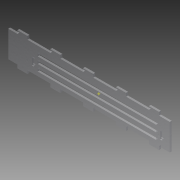
# Autodesk Inventor part: Panel3
Saved by Autodesk Inventor 2015 SP1 (Build 190203100, 203)
## iProperties
Created: 2014-08-06
Part Number: Panel3
Material: Acrylic, Clear
Document SubType Name: Modeling
Designer: Patrick Camilleri
Density: 1.19 g/cm^3
Appearance: Transparent - Clear
Author: Patrick Camilleri
Autodesk Inventor part; units mm, degrees
ref_plane "YZ Plane" through (0, 0, 0) normal (1, 0, 0) x (0, 1, 0)
ref_plane "XZ Plane" through (0, 0, 0) normal (0, 1, 0) x (-1, 0, 0)
ref_plane "XY Plane" through (0, 0, 0) normal (0, 0, 1) x (1, 0, 0)
sketch "Sketch1" plane through (0, 0, 0) normal (0, 1, 0) x (-1, 0, 0)
  line L0 (20.15, 134.75) -> (-20.15, 134.75)
  line L1 (-20.15, 134.75) -> (-20.15, -110.95)
  line L2 (-20.15, -110.95) -> (20.15, -110.95)
  line L3 (20.15, -110.95) -> (20.15, 134.75)
  line L4 (20.15, 0) -> (-20.15, 0) construction
  line L5 (0, -110.95) -> (0, 134.75) construction
  point P0 (0, 0)
  point P1 (0, 0)
  dimension "d57" = 40.3
  dimension "d58" = 110.95
  dimension "d59" = 134.75
  constraints: 12 end point, 3 midpoint, 2 parallel, 2 perpendicular, 2 point on line, 1 coincident, 1 horizontal
  measures "d57" distance of L1.end L2.end
  measures "d58" distance between parallel lines of L4 L2
  measures "d59" distance between parallel lines of L4 L0
extrude "Extrusion1" add sketch "Sketch1" along normal blind 3
sketch "Sketch3" plane through (0, 0, 0) normal (0, -1, 0) x (1, 0, 0)
  line L0 (20.15, -110.95) -> (-20.15, -110.95) projected
  line L1 (20.15, 134.75) -> (20.15, -110.95) projected
  line L2 (-20.15, -110.95) -> (-20.15, 134.75) projected
  line L3 (-25.15, -79.15) -> (-20.15, -79.15)
  line L4 (-20.15, -79.15) -> (-20.15, -94.45)
  line L5 (-20.15, -94.45) -> (-25.15, -94.45)
  line L6 (-25.15, -94.45) -> (-25.15, -79.15)
  line L7 (-25.15, -79.15) -> (-20.15, -94.45) construction
  line L8 (-20.15, -79.15) -> (-25.15, -94.45) construction
  line L9 (25.15, -94.45) -> (20.15, -94.45)
  line L10 (20.15, -94.45) -> (20.15, -79.15)
  line L11 (20.15, -79.15) -> (25.15, -79.15)
  line L12 (25.15, -79.15) -> (25.15, -94.45)
  line L13 (25.15, -94.45) -> (20.15, -79.15) construction
  line L14 (20.15, -94.45) -> (25.15, -79.15) construction
  point P0 (0, 0)
  point P1 (-22.65, -86.8)
  point P2 (22.65, -86.8)
  point P3 (20.15, -86.8)
  dimension "d61" = 15.3
  dimension "d64" = 5
  dimension "d65" = 15.3
  dimension "d78" = 24.15
  dimension "d79" = 24.15
  dimension "d97" = 5
  constraints: 24 end point, 5 midpoint, 4 parallel, 2 horizontal, 2 perpendicular, 2 point on line
  measures "d61" distance of L3.end L4.end
  measures "d64" distance of L10.end L11.end
  measures "d65" distance of L9.end L10.end
  measures "d78" distance from line of L0 point (-22.65, -86.8)
  measures "d79" distance from line of L0 point (22.65, -86.8)
  measures "d97" distance between parallel lines of L6 L4
extrude "Extrusion3" add sketch "Sketch3" against normal blind 3
pattern_linear "Rectangular Pattern1" count 5 spacing 50 along (0, 0, 1) of "Extrusion3"
sketch "Sketch4" plane through (0, 0, 0) normal (0, -1, 0) x (1, 0, 0)
  line L0 (20.15, -110.95) -> (-20.15, -110.95) projected
  line L1 (1, -96.15) -> (9, -96.15)
  line L2 (9, -96.15) -> (9, -98.85)
  line L3 (9, -98.85) -> (1, -98.85)
  line L4 (1, -98.85) -> (1, -96.15)
  line L5 (1, -96.15) -> (9, -98.85) construction
  line L6 (9, -96.15) -> (1, -98.85) construction
  line L7 (5, -118.696) -> (5, 153.6812) construction
  point P0 (5, -97.5)
  point P1 (5, -97.5)
  point P2 (5, -97.5)
  point P3 (5, -97.5)
  point P4 (0, 0)
  dimension "d69" = 8
  dimension "d70" = 2.7
  dimension "d98" = 13.45
  dimension "d100" = 5
  constraints: 14 end point, 4 midpoint, 2 parallel, 1 coincident, 1 horizontal, 1 perpendicular, 1 point on line, 1 vertical, 1 other
  measures "d69" distance of L2.end L3.end
  measures "d70" distance of L1.end L2.end
  measures "d98" distance from line of L0 point (5, -97.5)
  measures "d100" distance from line of point (0, 0) L7
extrude "Extrusion4" cut sketch "Sketch4" against normal blind 3
pattern_linear "Rectangular Pattern2" count 2 spacing 195 along (0, 0, 1) of "Extrusion4"
sketch "Sketch8" plane through (0, 3, 0) normal (0, 1, 0) x (1, 0, 0)
  line L0 (-10, -90) -> (-6, -90)
  line L1 (-6, -90) -> (-6, 90)
  line L2 (-6, 90) -> (-10, 90)
  line L3 (-10, 90) -> (-10, -90)
  line L4 (-10, -90) -> (-6, 90) construction
  line L5 (-6, -90) -> (-10, 90) construction
  point P0 (0, 0)
  point P1 (-8, 0)
  dimension "d82" = 4
  dimension "d83" = 180
  dimension "d84" = 6
  constraints: 12 end point, 2 midpoint, 2 parallel, 1 horizontal, 1 perpendicular
  measures "d82" distance of L2.end L1.end
  measures "d83" distance of L1.end L0.end
  measures "d84" distance from line of L1 point (0, 0)
extrude "Extrusion5" cut sketch "Sketch8" against normal through all
sketch "Sketch9" plane through (0, 3, 0) normal (0, 1, 0) x (1, 0, 0)
  line L0 (1, 96.15) -> (1, 98.85) projected
  line L1 (1, 98.85) -> (9, 98.85) projected
  line L2 (9, 98.85) -> (9, 96.15) projected
  line L3 (9, 96.15) -> (1, 96.15) projected
  line L4 (-0.35, 96.15) -> (10.35, 96.15)
  line L5 (10.35, 96.15) -> (10.35, 98.85)
  line L6 (10.35, 98.85) -> (-0.35, 98.85)
  line L7 (-0.35, 98.85) -> (-0.35, 96.15)
  line L8 (-0.35, 96.15) -> (10.35, 98.85) construction
  line L9 (10.35, 96.15) -> (-0.35, 98.85) construction
  line L10 (1, 98.85) -> (9, 96.15) construction
  line L11 (9, 96.15) -> (9, 98.85) construction
  line L12 (9, 98.85) -> (1, 96.15) construction
  point P0 (0, 0)
  point P1 (5, 97.5)
  point P2 (5, 97.5)
  dimension "d90" = 10.7
  dimension "d91" = 2.7
  constraints: 18 end point, 4 midpoint, 3 equal length, 1 horizontal, 1 perpendicular
  measures "d90" distance of L6.end L5.end
  measures "d91" distance of L5.end L4.end
extrude "Extrusion6" cut sketch "Sketch9" against normal blind 1.5 contours L4 L7 L6 L0 | L2 L6 L5 L4
pattern_linear "Rectangular Pattern4" count 2 spacing 195 along (0, 0, 1) of "Extrusion6"
pattern_linear "Rectangular Pattern5" count 3 spacing 10 along (1, 0, 0) of "Extrusion5"
equation "\"d79\" = d78"
equation "\"kerf\" = 0.15"
body "Solid1"
